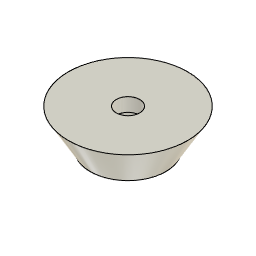
Tilt Tent Foot (Autodesk Fusion 360 design; units mm, degrees)
Autodesk Fusion 360 part; units mm, degrees
sketch "Sketch1" plane through (0, 0, 0) normal (0, 0, 1) x (1, 0, 0)
  circle A0 centre (0, 0) radius 5
  circle A1 centre (0, 0) radius 2.85
  circle A2 centre (0, 0) radius 1.55
  dimension "d1" = 10
  dimension "d2" = 5.7
  dimension "d5" = 3.1
  constraint coincident A0.centre A1.centre
  constraint concentric A0 A1
  constraint concentric A0 A2
  measures "d1" diameter of A0
  measures "d2" diameter of A1
  measures "d5" diameter of A2
extrude "Extrude1" add sketch "Sketch1" along normal blind 5 draft 30 contours A0 | A1 | A2
extrude "Extrude2" cut sketch "Sketch1" along normal blind 3.2 contours A1 | A2
extrude "Extrude3" cut sketch "Sketch1" along normal up to surface (5 mm away) contours A2
